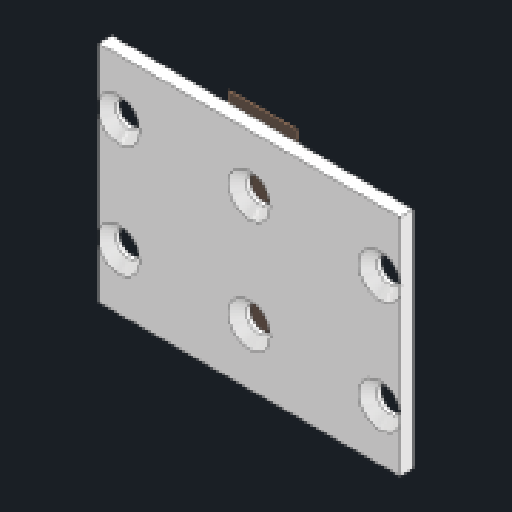
# Autodesk Inventor part: front_gear_holder
Saved by Autodesk Inventor 2023 (Build 270158000, 158)
## iProperties
Created: 2024-04-25
Part Number: front_gear_holder
Material: ABS Plastic
Document SubType Name: Modeling
Designer: szymo
Density: 1.06 g/cm^3
Appearance: Smooth - White
Author: szymo
Autodesk Inventor part; units mm, degrees
ref_plane "YZ Plane" through (0, 0, 0) normal (1, 0, 0) x (0, 1, 0)
ref_plane "XZ Plane" through (0, 0, 0) normal (0, 1, 0) x (-1, 0, 0)
ref_plane "Work Plane1" through (0, 0, 0) normal (0, 0, 1) x (1, 0, 0)
sketch "Sketch1" plane through (0, 0, 0) normal (0, 0, 1) x (1, 0, 0)
  line L0 (-12, 33.5) -> (-18, 33.5) projected
  line L1 (-18, 0) -> (-18, 33.5) projected
  line L2 (-18, 0) -> (-12, 0) projected
  line L3 (-12, 0) -> (-12, 33.5) projected
  line L4 (27, 33.5) -> (21, 33.5) projected
  line L5 (21, 0) -> (21, 33.5) projected
  line L6 (21, 0) -> (27, 0) projected
  line L7 (27, 0) -> (27, 33.5) projected
  line L8 (-18, 33.5) -> (27, 33.5)
  line L9 (27, 33.5) -> (27, 0)
  line L10 (27, 0) -> (-18, 0)
  line L11 (-18, 0) -> (-18, 33.5)
  circle A0 centre (-15, 25.125) radius 2.3 projected
  circle A1 centre (-15, 8.375) radius 2.3 projected
  circle A2 centre (24, 24.4375) radius 2.3 projected
  circle A3 centre (24, 7.6875) radius 2.3 projected
  point P0 (0, 0)
  constraints: 8 end point, 2 parallel, 1 horizontal, 1 perpendicular
ref_plane "Work Plane2" through (-69.2, 0, 2) normal (0, 0, -1) x (0, 1, 0)
extrude "Extrusion1" add sketch "Sketch1" along normal up to surface (2 mm away) contours L3 L2 L1 L0 | L8 L5 L10 L3 | L4 L7 L6 L5 | A0 | A1 | A2 | A3
sketch "Sketch2" plane through (-18, 33.5, 2) normal (0, 0, 1) x (1, 0, 0)
  circle A0 centre (3, -8.375) radius 2.3 projected
  circle A1 centre (3, -25.125) radius 2.3 projected
  line L0 (6, 0) -> (0, 0) projected
  line L1 (0, -33.5) -> (0, 0) projected
  line L2 (0, -33.5) -> (6, -33.5) projected
  line L3 (6, -33.5) -> (6, 0) projected
  circle A2 centre (22.5, -25.125) radius 2.3 projected
  circle A3 centre (22.5, -8.375) radius 2.3 projected
  line L4 (27, 0) -> (18, 0) projected
  line L5 (18, -33.5) -> (18, 0) projected
  line L6 (18, -33.5) -> (27, -33.5) projected
  line L7 (27, -33.5) -> (27, 0) projected
  circle A4 centre (42, -9.0625) radius 2.3 projected
  circle A5 centre (42, -25.8125) radius 2.3 projected
  line L8 (45, 0) -> (39, 0) projected
  line L9 (39, -33.5) -> (39, 0) projected
  line L10 (39, -33.5) -> (45, -33.5) projected
  line L11 (45, -33.5) -> (45, 0) projected
hole "Hole1" at (-15, 25.125, 2) at (-15, 8.375, 2) at (4.5, 8.375, 2) at (4.5, 25.125, 2) at (24, 24.4375, 2) at (24, 7.6875, 2) direction (0, 0, -1) diameter 3.6 end through all countersink diameter 6.3 countersink angle 90 clearance for "Countersunk Flat Head Screw ISO 2009/7046" size "M3" standard "ISO"
body "Solid1"
